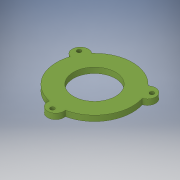
# Autodesk Inventor part: HarmonicDrive
Saved by Autodesk Inventor 2018.3 (Build 223284000, 284)
## iProperties
Created: 2018-06-22
Part Number: HarmonicDrive
Material: Generisch
Document SubType Name: Modeling
Designer: JochenAlt
Density: 1 g/cm^3
Appearance: Vorgabe
Author: JochenAlt
Autodesk Inventor part; units mm, degrees
ref_plane "YZ Plane" through (0, 0, 0) normal (1, 0, 0) x (0, 1, 0)
ref_plane "XZ Plane" through (0, 0, 0) normal (0, 1, 0) x (-1, 0, 0)
sketch "Riemen" plane through (0, 0, 0) normal (0, 0, 1) x (1, 0, 0)
  circle A0 centre (0, 0) radius 19.0986 construction
  circle A1 centre (0, 0) radius 17.3586
  circle A2 centre (0, 0) radius 21.1586 construction
  line L0 (0, 250.5339) -> (0, -318.2557) construction
  line L1 (-30.0896, 0) -> (30.0896, 0) construction
  line L2 (0, 0) -> (6.228, 23.2432) construction
  arc A3 (5.4762, 20.4376) -> (3.6141, 19.1985) centre (5.0906, 18.9984) ccw
  arc A4 (1.478, 19.4797) -> (1.8538, 19.0084) centre (1.8946, 19.4264) ccw
  arc A5 (3.1291, 18.8405) -> (3.6141, 19.1985) centre (3.1979, 19.2548) ccw
  line L3 (1.8538, 19.0084) -> (3.1291, 18.8405)
  arc A6 (1.478, 19.4797) -> (0, 21.1586) centre (0, 19.6686) ccw
  arc A7 (-3.6141, 19.1985) -> (-5.4762, 20.4376) centre (-5.0906, 18.9984) ccw
  arc A8 (-3.6141, 19.1985) -> (-3.1291, 18.8405) centre (-3.1979, 19.2548) ccw
  line L4 (-3.1291, 18.8405) -> (-1.8538, 19.0084)
  arc A9 (-1.8538, 19.0084) -> (-1.478, 19.4797) centre (-1.8946, 19.4264) ccw
  arc A10 (0, 21.1586) -> (-1.478, 19.4797) centre (0, 19.6686) ccw
  arc A11 (-8.4599, 17.6089) -> (-10.5793, 18.3239) centre (-9.8343, 17.0335) ccw
  arc A12 (-8.4599, 17.6089) -> (-7.8988, 17.3887) centre (-8.0725, 17.7711) ccw
  line L5 (-7.8988, 17.3887) -> (-6.7104, 17.8809)
  arc A13 (-6.7104, 17.8809) -> (-6.4693, 18.4334) centre (-6.858, 18.2741) ccw
  arc A14 (-5.4762, 20.4376) -> (-6.4693, 18.4334) centre (-5.0906, 18.9984) ccw
  arc A15 (-12.7291, 14.8193) -> (-14.9614, 14.9614) centre (-13.9078, 13.9078) ccw
  arc A16 (-12.7291, 14.8193) -> (-12.1301, 14.7518) centre (-12.3969, 15.0762) ccw
  line L6 (-12.1301, 14.7518) -> (-11.1097, 15.5349)
  arc A17 (-11.1097, 15.5349) -> (-11.0198, 16.1309) centre (-11.354, 15.8765) ccw
  arc A18 (-10.5793, 18.3239) -> (-11.0198, 16.1309) centre (-9.8343, 17.0335) ccw
  arc A19 (-16.1309, 11.0198) -> (-18.3239, 10.5793) centre (-17.0335, 9.8343) ccw
  arc A20 (-16.1309, 11.0198) -> (-15.5349, 11.1097) centre (-15.8765, 11.354) ccw
  line L7 (-15.5349, 11.1097) -> (-14.7518, 12.1301)
  arc A21 (-14.7518, 12.1301) -> (-14.8193, 12.7291) centre (-15.0762, 12.3969) ccw
  arc A22 (-14.9614, 14.9614) -> (-14.8193, 12.7291) centre (-13.9078, 13.9078) ccw
  arc A23 (-18.4334, 6.4693) -> (-20.4376, 5.4762) centre (-18.9984, 5.0906) ccw
  arc A24 (-18.4334, 6.4693) -> (-17.8809, 6.7104) centre (-18.2741, 6.858) ccw
  line L8 (-17.8809, 6.7104) -> (-17.3887, 7.8988)
  arc A25 (-17.3887, 7.8988) -> (-17.6089, 8.4599) centre (-17.7711, 8.0725) ccw
  arc A26 (-18.3239, 10.5793) -> (-17.6089, 8.4599) centre (-17.0335, 9.8343) ccw
  arc A27 (-19.4797, 1.478) -> (-21.1586, 0) centre (-19.6686, 0) ccw
  arc A28 (-19.4797, 1.478) -> (-19.0084, 1.8538) centre (-19.4264, 1.8946) ccw
  line L9 (-19.0084, 1.8538) -> (-18.8405, 3.1291)
  arc A29 (-18.8405, 3.1291) -> (-19.1985, 3.6141) centre (-19.2548, 3.1979) ccw
  arc A30 (-20.4376, 5.4762) -> (-19.1985, 3.6141) centre (-18.9984, 5.0906) ccw
  arc A31 (-19.1985, -3.6141) -> (-20.4376, -5.4762) centre (-18.9984, -5.0906) ccw
  arc A32 (-19.1985, -3.6141) -> (-18.8405, -3.1291) centre (-19.2548, -3.1979) ccw
  line L10 (-18.8405, -3.1291) -> (-19.0084, -1.8538)
  arc A33 (-19.0084, -1.8538) -> (-19.4797, -1.478) centre (-19.4264, -1.8946) ccw
  arc A34 (-21.1586, 0) -> (-19.4797, -1.478) centre (-19.6686, 0) ccw
  arc A35 (-17.6089, -8.4599) -> (-18.3239, -10.5793) centre (-17.0335, -9.8343) ccw
  arc A36 (-17.6089, -8.4599) -> (-17.3887, -7.8988) centre (-17.7711, -8.0725) ccw
  line L11 (-17.3887, -7.8988) -> (-17.8809, -6.7104)
  arc A37 (-17.8809, -6.7104) -> (-18.4334, -6.4693) centre (-18.2741, -6.858) ccw
  arc A38 (-20.4376, -5.4762) -> (-18.4334, -6.4693) centre (-18.9984, -5.0906) ccw
  arc A39 (-14.8193, -12.7291) -> (-14.9614, -14.9614) centre (-13.9078, -13.9078) ccw
  arc A40 (-14.8193, -12.7291) -> (-14.7518, -12.1301) centre (-15.0762, -12.3969) ccw
  line L12 (-14.7518, -12.1301) -> (-15.5349, -11.1097)
  arc A41 (-15.5349, -11.1097) -> (-16.1309, -11.0198) centre (-15.8765, -11.354) ccw
  arc A42 (-18.3239, -10.5793) -> (-16.1309, -11.0198) centre (-17.0335, -9.8343) ccw
  arc A43 (-11.0198, -16.1309) -> (-10.5793, -18.3239) centre (-9.8343, -17.0335) ccw
  arc A44 (-11.0198, -16.1309) -> (-11.1097, -15.5349) centre (-11.354, -15.8765) ccw
  line L13 (-11.1097, -15.5349) -> (-12.1301, -14.7518)
  arc A45 (-12.1301, -14.7518) -> (-12.7291, -14.8193) centre (-12.3969, -15.0762) ccw
  arc A46 (-14.9614, -14.9614) -> (-12.7291, -14.8193) centre (-13.9078, -13.9078) ccw
  arc A47 (-6.4693, -18.4334) -> (-5.4762, -20.4376) centre (-5.0906, -18.9984) ccw
  arc A48 (-6.4693, -18.4334) -> (-6.7104, -17.8809) centre (-6.858, -18.2741) ccw
  line L14 (-6.7104, -17.8809) -> (-7.8988, -17.3887)
  arc A49 (-7.8988, -17.3887) -> (-8.4599, -17.6089) centre (-8.0725, -17.7711) ccw
  arc A50 (-10.5793, -18.3239) -> (-8.4599, -17.6089) centre (-9.8343, -17.0335) ccw
  arc A51 (-1.478, -19.4797) -> (0, -21.1586) centre (0, -19.6686) ccw
  arc A52 (-1.478, -19.4797) -> (-1.8538, -19.0084) centre (-1.8946, -19.4264) ccw
  line L15 (-1.8538, -19.0084) -> (-3.1291, -18.8405)
  arc A53 (-3.1291, -18.8405) -> (-3.6141, -19.1985) centre (-3.1979, -19.2548) ccw
  arc A54 (-5.4762, -20.4376) -> (-3.6141, -19.1985) centre (-5.0906, -18.9984) ccw
  arc A55 (3.6141, -19.1985) -> (5.4762, -20.4376) centre (5.0906, -18.9984) ccw
  arc A56 (3.6141, -19.1985) -> (3.1291, -18.8405) centre (3.1979, -19.2548) ccw
  line L16 (3.1291, -18.8405) -> (1.8538, -19.0084)
  arc A57 (1.8538, -19.0084) -> (1.478, -19.4797) centre (1.8946, -19.4264) ccw
  arc A58 (0, -21.1586) -> (1.478, -19.4797) centre (0, -19.6686) ccw
  arc A59 (8.4599, -17.6089) -> (10.5793, -18.3239) centre (9.8343, -17.0335) ccw
  arc A60 (8.4599, -17.6089) -> (7.8988, -17.3887) centre (8.0725, -17.7711) ccw
  line L17 (7.8988, -17.3887) -> (6.7104, -17.8809)
  arc A61 (6.7104, -17.8809) -> (6.4693, -18.4334) centre (6.858, -18.2741) ccw
  arc A62 (5.4762, -20.4376) -> (6.4693, -18.4334) centre (5.0906, -18.9984) ccw
  arc A63 (12.7291, -14.8193) -> (14.9614, -14.9614) centre (13.9078, -13.9078) ccw
  arc A64 (12.7291, -14.8193) -> (12.1301, -14.7518) centre (12.3969, -15.0762) ccw
  line L18 (12.1301, -14.7518) -> (11.1097, -15.5349)
  arc A65 (11.1097, -15.5349) -> (11.0198, -16.1309) centre (11.354, -15.8765) ccw
  arc A66 (10.5793, -18.3239) -> (11.0198, -16.1309) centre (9.8343, -17.0335) ccw
  arc A67 (16.1309, -11.0198) -> (18.3239, -10.5793) centre (17.0335, -9.8343) ccw
  arc A68 (16.1309, -11.0198) -> (15.5349, -11.1097) centre (15.8765, -11.354) ccw
  line L19 (15.5349, -11.1097) -> (14.7518, -12.1301)
  arc A69 (14.7518, -12.1301) -> (14.8193, -12.7291) centre (15.0762, -12.3969) ccw
  arc A70 (14.9614, -14.9614) -> (14.8193, -12.7291) centre (13.9078, -13.9078) ccw
  arc A71 (18.4334, -6.4693) -> (20.4376, -5.4762) centre (18.9984, -5.0906) ccw
  arc A72 (18.4334, -6.4693) -> (17.8809, -6.7104) centre (18.2741, -6.858) ccw
  line L20 (17.8809, -6.7104) -> (17.3887, -7.8988)
  arc A73 (17.3887, -7.8988) -> (17.6089, -8.4599) centre (17.7711, -8.0725) ccw
  arc A74 (18.3239, -10.5793) -> (17.6089, -8.4599) centre (17.0335, -9.8343) ccw
  arc A75 (19.4797, -1.478) -> (21.1586, 0) centre (19.6686, 0) ccw
  arc A76 (19.4797, -1.478) -> (19.0084, -1.8538) centre (19.4264, -1.8946) ccw
  line L21 (19.0084, -1.8538) -> (18.8405, -3.1291)
  arc A77 (18.8405, -3.1291) -> (19.1985, -3.6141) centre (19.2548, -3.1979) ccw
  arc A78 (20.4376, -5.4762) -> (19.1985, -3.6141) centre (18.9984, -5.0906) ccw
  arc A79 (19.1985, 3.6141) -> (20.4376, 5.4762) centre (18.9984, 5.0906) ccw
  arc A80 (19.1985, 3.6141) -> (18.8405, 3.1291) centre (19.2548, 3.1979) ccw
  line L22 (18.8405, 3.1291) -> (19.0084, 1.8538)
  arc A81 (19.0084, 1.8538) -> (19.4797, 1.478) centre (19.4264, 1.8946) ccw
  arc A82 (21.1586, 0) -> (19.4797, 1.478) centre (19.6686, 0) ccw
  arc A83 (17.6089, 8.4599) -> (18.3239, 10.5793) centre (17.0335, 9.8343) ccw
  arc A84 (17.6089, 8.4599) -> (17.3887, 7.8988) centre (17.7711, 8.0725) ccw
  line L23 (17.3887, 7.8988) -> (17.8809, 6.7104)
  arc A85 (17.8809, 6.7104) -> (18.4334, 6.4693) centre (18.2741, 6.858) ccw
  arc A86 (20.4376, 5.4762) -> (18.4334, 6.4693) centre (18.9984, 5.0906) ccw
  arc A87 (14.8193, 12.7291) -> (14.9614, 14.9614) centre (13.9078, 13.9078) ccw
  arc A88 (14.8193, 12.7291) -> (14.7518, 12.1301) centre (15.0762, 12.3969) ccw
  line L24 (14.7518, 12.1301) -> (15.5349, 11.1097)
  arc A89 (15.5349, 11.1097) -> (16.1309, 11.0198) centre (15.8765, 11.354) ccw
  arc A90 (18.3239, 10.5793) -> (16.1309, 11.0198) centre (17.0335, 9.8343) ccw
  arc A91 (11.0198, 16.1309) -> (10.5793, 18.3239) centre (9.8343, 17.0335) ccw
  arc A92 (11.0198, 16.1309) -> (11.1097, 15.5349) centre (11.354, 15.8765) ccw
  line L25 (11.1097, 15.5349) -> (12.1301, 14.7518)
  arc A93 (12.1301, 14.7518) -> (12.7291, 14.8193) centre (12.3969, 15.0762) ccw
  arc A94 (14.9614, 14.9614) -> (12.7291, 14.8193) centre (13.9078, 13.9078) ccw
  arc A95 (6.4693, 18.4334) -> (5.4762, 20.4376) centre (5.0906, 18.9984) ccw
  arc A96 (6.4693, 18.4334) -> (6.7104, 17.8809) centre (6.858, 18.2741) ccw
  line L26 (6.7104, 17.8809) -> (7.8988, 17.3887)
  arc A97 (7.8988, 17.3887) -> (8.4599, 17.6089) centre (8.0725, 17.7711) ccw
  arc A98 (10.5793, 18.3239) -> (8.4599, 17.6089) centre (9.8343, 17.0335) ccw
  dimension "d0" = 15
  dimension "d2" = 2.06
  dimension "d3" = 3.8
  dimension "d5" = 38.1972
  dimension "d6" = 0.42
  dimension "d7" = 1.49
  constraints: 194 point on circle, 98 centre point, 50 end point, 4 point on line, 4 tangent, 3 coincident, 2 equal radius, 1 vertical alignment, 3 other
  measures "d0" angle of L2 L0
  measures "d5" diameter of A0
  measures "d6" radius of A4
  measures "d7" radius of A6
sketch "Enclosure" plane through (0, 0, 0) normal (0, 0, 1) x (1, 0, 0)
  circle A0 centre (0, 0) radius 17.25
  circle A1 centre (0, 0) radius 27.5
  circle A2 centre (0, 0) radius 15.25
  circle A3 centre (0, 0) radius 25.5
  line L0 (0, 250.5339) -> (0, -318.2557) construction
  circle A4 centre (0, -30.5) radius 1.5
  circle A5 centre (-26.4138, 15.25) radius 1.5
  circle A6 centre (26.4138, 15.25) radius 1.5
  circle A7 centre (0, 0) radius 30.5 construction
  line L1 (5.3307, -24.9366) -> (5.7488, -26.8924) construction
  line L2 (-5.3307, -24.9366) -> (-5.7488, -26.8924) construction
  circle A8 centre (26.4138, 15.25) radius 2.5
  circle A9 centre (-26.4138, 15.25) radius 2.5
  circle A10 centre (0, -30.5) radius 2.5
  line L3 (0, 0) -> (-26.4138, 15.25) construction
  line L4 (26.4138, 15.25) -> (0, 0) construction
  arc A11 (-5.7488, -26.8924) -> (5.7488, -26.8924) centre (0, -28.1213) ccw
  line L5 (0, -33) -> (0, -34) construction
  arc A12 (-20.4151, 18.4248) -> (-26.1639, 8.4676) centre (-24.3538, 14.0607) ccw
  line L6 (-20.4151, 18.4248) -> (-18.9304, 17.0848) construction
  line L7 (-26.1639, 8.4676) -> (-24.2611, 7.8518) construction
  arc A13 (26.1639, 8.4676) -> (20.4151, 18.4248) centre (24.3538, 14.0607) ccw
  circle A14 centre (0, 0) radius 28.1213 construction
  circle A15 centre (0, 0) radius 10.75
  dimension "d101" = 5
  dimension "d12" = 55
  dimension "d13" = 34.5
  dimension "d14" = 30.5
  dimension "d19" = 2
  dimension "d35" = 3
  dimension "d36" = 3
  dimension "d181" = 1
  dimension "d182" = 120
  dimension "d191" = 21.5
  dimension "d22" = 21
  dimension "d23" = 19
  dimension "d45" = 12
  dimension "d218" = 30
  dimension "d239" = 20
  dimension "d240" = 1
  dimension "d241" = 1
  dimension "d47" = 12
  dimension "d48" = 3
  dimension "d51" = 2
  constraints: 22 point on circle, 15 centre point, 14 end point, 10 coincident, 6 point on line, 5 equal radius, 4 tangent, 1 vertical alignment, 4 other
  measures "d12" diameter of A1
  measures "d13" diameter of A0
  measures "d14" diameter of A2
  measures "d19" radial gap between concentric circles of A1 A3
  measures "d35" diameter of A4
  measures "d36" radial gap between concentric circles of A7 A1
  measures "d181" distance of L5.end L5.start
  measures "d182" angle of L4 L3
  measures "d191" diameter of A15
extrude "Extrusion1" add sketch "Enclosure" along normal blind 4 contours A0 | A1 | A3
extrude "Extrusion7" add sketch "Enclosure" along normal up to surface (4 mm away) contours A0 | A1 | A1 A13 | A11 A1 | A1 A12 | A3 | A8 | A9 | A10
extrude "Extrusion2" cut sketch "Riemen" along normal blind 3
sketch "Skizze7" plane through (0, 0, 0) normal (0, 1, 0) x (-1, 0, 0)
  line L0 (9, -63) -> (11.9916, -63)
  arc A0 (11.9916, -63) -> (27.5, -47.4916) centre (11.9916, -47.4916) ccw
  line L1 (26.0805, 0) -> (26.0805, -33) construction
  arc A1 (11.9916, -61) -> (25.5, -47.4916) centre (11.9916, -47.4916) ccw
  line L2 (11.9916, -61) -> (9, -61)
  line L3 (0, -214.7485) -> (0, 112.4908) construction
  line L4 (-16.9424, 0) -> (38.6543, 0) construction
  line L5 (9, -57) -> (9, -63) construction
  line L6 (9, -63) -> (9, -61)
  line L7 (-9, -63) -> (9, -63) construction
  line L8 (27.5, -47.4916) -> (27.5, -34)
  line L9 (27.5, -34) -> (25.5, -34)
  line L10 (25.5, -34) -> (25.5, -47.4916)
  line L11 (27.5, 0) -> (27.5, -32) construction
  line L12 (20.4151, -34) -> (30.2325, -34) construction
  point P0 (0, 0)
  point P1 (26.1639, -34)
  dimension "d93" = 2
  dimension "d123" = 32
  constraints: 26 end point, 6 perpendicular, 4 equal length, 3 point on circle, 1 centre point, 1 coincident, 1 collinear, 1 midpoint, 1 parallel, 1 point on line, 1 other
  measures "d123" distance of L2.start L2.end
sketch "Skizze9" plane through (0, 0, -48.5) normal (0, 0, 1) x (0.9999991, 0.0013544, 0)
  line L0 (-15.9533, 34.4925) -> (16.0467, 34.4491) projected
  line L1 (-15.9875, 9.2593) -> (-15.9533, 34.4925) projected
  line L2 (16.0467, 34.4491) -> (16.0125, 9.2159) projected
  line L3 (37.848, -3.4303) -> (21.8105, -31.1214) projected
  line L4 (-21.8947, -31.0622) -> (-37.8572, -3.3277) projected
  line L5 (-21.8947, -31.0622) -> (-0.025, -18.4752) projected
  line L6 (-37.8572, -3.3277) -> (-15.9875, 9.2593) projected
  line L7 (21.8105, -31.1214) -> (-0.025, -18.4752) projected
  line L8 (37.848, -3.4303) -> (16.0125, 9.2159) projected
  circle A0 centre (0, 0) radius 18.4752 projected
  dimension "d165" = 3
  dimension "d176" = 5
  dimension "d177" = 74
  dimension "d186" = 200
  dimension "d187" = 41
  dimension "d201" = 84.0923
  dimension "d203" = 84.0923
  dimension "d219" = 41
  dimension "d220" = 2
  dimension "d171" = 120
  dimension "d193" = 83
  dimension "d238" = 2
  dimension "d246" = 20
  dimension "d247" = 2
  dimension "d248" = 2
  constraints: 9 point on circle, 8 end point, 5 centre point, 3 coincident, 2 concentric, 2 point on line, 1 symmetric about line, 2 other
  measures "d171" angle of L2 L1
  measures "d238" distance of L3.start L3.end
  measures "d246" distance of L4.start L3.end
